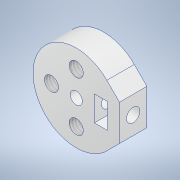
# Autodesk Inventor part: Wheel Hub
Saved by Autodesk Inventor 2022 (Build 260153000, 153)
## iProperties
Created: 2022-08-21
Part Number: Wheel Hub
Material: Aluminum 6061
Document SubType Name: Modeling
Designer: Nick
Density: 2.7 g/cm^3
Appearance: Aluminum - Flat
Mass: 3.97923 g
Surface Area: 12.9976 cm^2
Volume: 1.47379 cm^3
Author: Nick
Autodesk Inventor part; units mm, degrees
ref_plane "YZ Plane" through (0, 0, 0) normal (1, 0, 0) x (0, 1, 0)
ref_plane "XZ Plane" through (0, 0, 0) normal (0, 1, 0) x (-1, 0, 0)
ref_plane "XY Plane" through (0, 0, 0) normal (0, 0, 1) x (1, 0, 0)
sketch "Sketch1" plane through (0, 0, 0) normal (0, 0, 1) x (1, 0, 0)
  circle A0 centre (0, 0) radius 1.4
  circle A1 centre (0, 0) radius 10
  line L0 (7.0711, 7.0711) -> (10, 4.1421)
  line L1 (10, 4.1421) -> (10, -4.1421)
  line L2 (10, -4.1421) -> (7.0711, -7.0711)
  point P0 (10, 0)
  point P1 (10, 0)
  point P2 (10, 0)
  dimension "d0" = 2.8
  dimension "d1" = 20
  dimension "d33" = 135
  constraints: 6 end point, 3 tangent, 2 centre point, 2 coincident, 2 horizontal alignment, 2 point on circle, 1 midpoint, 1 vertical
  measures "d0" diameter of A0
  measures "d1" diameter of A1
  measures "d33" angle of L1 L0
extrude "Extrusion1" add sketch "Sketch1" along normal blind 6.35
sketch "Sketch2" plane through (0, 0, 6.35) normal (0, 0, 1) x (0, -1, 0)
  arc A0 (-7.0711, 7.0711) -> (7.0711, 7.0711) centre (0, 0) ccw projected
  circle A1 centre (0, 0) radius 1.4 projected
  line L0 (-1.7564, 1.4) -> (1.7564, 1.4) construction
  line L1 (-0.2885, 10) -> (0.2885, 10) construction
  line L2 (4.1421, 10) -> (-4.1421, 10) projected
  line L3 (-1.5, -10) -> (1.5, -10)
  point P0 (0, -5.75)
  point P1 (0, 10)
  point P2 (0, 1.4)
  point P3 (0, -10)
  dimension "d34" = 4.25
  constraints: 6 end point, 4 midpoint, 3 horizontal, 3 vertical alignment, 1 point on circle, 1 tangent
  measures "d34" distance from line of point (0, -5.75) L3
hole "Hole1" at (-5.75, 0, 6.35) direction (0, 0, -1) diameter 3.242 end through all thread size "M4x0.7" class "6H" standard "ANSI Metric M Profile"
pattern_circular "Circular Pattern1" count 4 over 360 about axis through (0, 0, 0) along (0, 0, 1) of "Hole1" skipped copies 3
sketch "Sketch5" plane through (0, 0, 6.35) normal (0, 0, 1) x (1, 0, 0)
  circle A0 centre (0, 0) radius 1.4 projected
  line L0 (4.2, 2.9) -> (7.2, 2.9)
  line L1 (7.2, 2.9) -> (7.2, -2.9)
  line L2 (7.2, -2.9) -> (4.2, -2.9)
  line L3 (4.2, -2.9) -> (4.2, 2.9)
  line L4 (10, -4.1421) -> (10, 4.1421) projected
  circle A1 centre (0, 0) radius 1.4 projected
  line L5 (1.4, 0) -> (10, 0)
  point P0 (5.7, 2.9)
  point P1 (5.7, 0)
  point P2 (5.7, 0)
  point P3 (5.7, 0)
  point P4 (7.2, 0)
  dimension "d28" = 5.8
  dimension "d29" = 3
  constraints: 10 end point, 4 midpoint, 3 horizontal alignment, 2 coincident, 2 parallel, 1 horizontal, 1 perpendicular, 1 vertical alignment, 1 other
  measures "d28" distance of L0.end L1.end
  measures "d29" distance of L0.start L0.end
extrude "Extrusion3" cut sketch "Sketch5" against normal blind 10 contours L0 L1 L5 L3 | L5 L1 L2 L3
sketch "Sketch6" plane through (10, -4.1421, 0) normal (1, 0, 0) x (0, 0, -1)
  line L0 (0, 0) -> (0, 8.2843) projected
  line L1 (0, 8.2843) -> (-6.35, 8.2843) projected
  point P0 (0, 4.1421)
  point P1 (-3.175, 4.1421)
  point P2 (0, 4.1421)
  point P3 (-3.175, 8.2843)
  constraints: 2 midpoint, 1 horizontal alignment, 1 vertical alignment
hole "Hole3" at (10, 0, 3.175) direction (-1, 0, 0) diameter 3.1 depth 10 clearance for "Flat Head Machine Screw" size "M3" standard "Ansi Metric M Profile"
body "Solid1"
